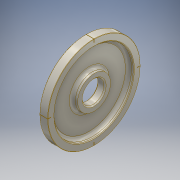
# Autodesk Inventor part: Wheel
Saved by Autodesk Inventor 2016 (Build 200138000, 138)
## iProperties
Created: 2021-04-07
Part Number: Wheel
Material: Типовые
Document SubType Name: Modeling
Designer: Лол
Density: 1 g/cm^3
Appearance: Титан
Mass: 170.452 g
Surface Area: 559.096 cm^2
Volume: 170.452 cm^3
Author: Лол
Autodesk Inventor part; units mm, degrees
ref_plane "YZ Plane" through (0, 0, 0) normal (1, 0, 0) x (0, 1, 0)
ref_plane "XZ Plane" through (0, 0, 0) normal (0, 1, 0) x (-1, 0, 0)
ref_plane "XY Plane" through (0, 0, 0) normal (0, 0, 1) x (1, 0, 0)
sketch "Эскиз1" plane through (0, 0, 0) normal (0, 0, 1) x (1, 0, 0)
  line L0 (0, 20) -> (0, 30)
  line L1 (1, 30.1228) -> (1, 72.3772)
  line L2 (0, 72.5) -> (0, 84.4165)
  line L3 (0, 84.4165) -> (15, 84.4165)
  line L4 (6, 71.3949) -> (6, 31.1051)
  line L5 (15, 20) -> (0, 20)
  line L6 (15, 30) -> (15, 20)
  line L7 (-3, 0) -> (18, 0) construction
  line L8 (0, -16.8833) -> (0, 101.2998) construction
  line L9 (15, 84.4165) -> (15, 72.5)
  line L10 (15, 72.5) -> (6, 71.3949)
  line L11 (15, 30) -> (6, 31.1051)
  line L12 (0, 30) -> (1, 30.1228)
  line L13 (0, 72.5) -> (1, 72.3772)
  point P0 (0, 0)
  point P1 (1, 77.4165)
  point P2 (7, 77.4165)
  point P3 (7, 28)
  dimension "d0" = 15
  dimension "d2" = 5
  dimension "d5" = 40
  dimension "d7" = 168.833
  dimension "d9" = 0
  dimension "d17" = 83
  dimension "d18" = 83
  dimension "d19" = 60
  dimension "d20" = 83
  dimension "d21" = 83
  dimension "d22" = 2
  dimension "d43" = 145
  constraints: 24 end point, 4 parallel, 3 point on line, 2 perpendicular, 1 vertical
  measures "d0" distance of L2.end L3.end
  measures "d2" distance between parallel lines of L4 L1
  measures "d5" diameter of L5 L7
  measures "d7" diameter of L3 L7
  measures "d9" distance between parallel lines of L0 L8
  measures "d17" angle of L4 L10
  measures "d18" angle of L11 L4
  measures "d19" diameter of L6.start L7
  measures "d20" angle of L1 L13
  measures "d21" angle of L12 L1
  measures "d22" diameter of L1 L8
  measures "d43" diameter of L9.end L7
revolve "Вращение1" add sketch "Эскиз1" angle 360 about axis through (-10, 0, 0) along (1, 0, 0)
chamfer "Фаска1" distance 2 angle 45 2 edges at (15, -20, 0) (0, -20, 0)
fillet "Сопряжение3" radius 6 2 edges at (6, -71.3949, 0) (6, -31.1051, 0)
chamfer "Фаска2" distance 1 angle 45 1 edges at (15, -72.5, 0)
fillet "Сопряжение4" radius 6 2 edges at (1, -30.1228, 0) (1, -72.3772, 0)
chamfer "Фаска4" distance 0.5 angle 45 2 edges at (0, -84.4165, 0) (15, -84.4165, 0)
sketch "Эскиз2" plane through (15, 0, 0) normal (1, 0, 0) x (0, 0, -1)
  circle A0 centre (0, 0) radius 84.4165 projected
  circle A1 centre (0, 0) radius 73.5 projected
  circle A2 centre (0, 0) radius 84.4165 projected
  line L0 (-84.4161, 0.25) -> (-78.79, 0.25)
  line L1 (-78.79, 0.25) -> (-78.79, -0.25)
  line L2 (-78.79, -0.25) -> (-84.4161, -0.25)
  line L3 (0, -118.1831) -> (0, 118.1831) projected
  line L4 (118.1831, 0) -> (-118.1831, 0) projected
  dimension "d33" = 78.79
  dimension "d34" = 0.5
  constraints: 6 end point, 4 point on circle, 1 horizontal, 1 perpendicular, 1 other
  measures "d33" distance between parallel lines of L3 L1
  measures "d34" distance between parallel lines of L2 L0
extrude "Выдавливание1" cut sketch "Эскиз2" against normal through all contours L0 L1 L4 A0 | A0 L4 L1 L2
pattern_circular "Круговой массив1" count 4 over 360 about axis through (-10, 0, 0) along (1, 0, 0) of "Выдавливание1"
